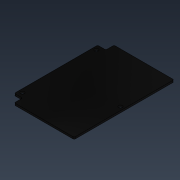
# Autodesk Inventor part: Base Station PCB
Saved by Autodesk Inventor 2022.1 (Build 261234020, 234B)
## iProperties
Created: 2017-10-12
Part Number: Base Station PCB
Material: Phenolharz
Document SubType Name: Modeling
Designer: ryll
Density: 1.38 g/cm^3
Appearance: Glänzend - Schwarz
Mass: 15.8976 g
Surface Area: 149.895 cm^2
Volume: 11.52 cm^3
Author: ryll
Autodesk Inventor part; units mm, degrees
ref_plane "YZ Plane" through (0, 0, 0) normal (1, 0, 0) x (0, 1, 0)
ref_plane "XZ Plane" through (0, 0, 0) normal (0, 1, 0) x (-1, 0, 0)
ref_plane "XY Plane" through (0, 0, 0) normal (0, 0, 1) x (1, 0, 0)
sketch "Skizze1" plane through (0, 0, 0) normal (0, 0, 1) x (1, 0, 0)
  line L0 (-22, -42.5) -> (29, -42.5)
  line L1 (29, -42.5) -> (29, 42.5)
  line L2 (29, 42.5) -> (-22, 42.5)
  line L3 (-29, 35.5) -> (-29, -35.5)
  line L4 (-22, -42.5) -> (-22, -35.5)
  line L5 (-22, -35.5) -> (-29, -35.5)
  line L6 (-22, 42.5) -> (-22, 35.5)
  line L7 (-22, 35.5) -> (-29, 35.5)
  line L8 (0, 59.5) -> (0, -59.5) projected
  line L9 (-40.6, 0) -> (40.6, 0) projected
  dimension "d22" = 58
  dimension "d23" = 85
  dimension "d24" = 7
  dimension "d25" = 7
  dimension "d26" = 7
  dimension "d27" = 7
  constraints: 16 end point, 3 horizontal, 2 parallel, 2 vertical, 1 perpendicular, 2 other
  measures "d22" distance between parallel lines of L1 L3
  measures "d23" distance of L0.end L1.end
  measures "d24" distance of L6.end L3.start
  measures "d25" distance of L2.end L6.end
  measures "d26" distance of L4.end L3.end
  measures "d27" distance of L0.start L4.end
extrude "Extrusion1" add sketch "Skizze1" along normal blind 1.6
sketch "Skizze2" plane through (0, 0, 1.6) normal (0, 0, 1) x (1, 0, 0)
  line L0 (-22, -42.5) -> (29, -42.5) projected
  line L1 (29, -42.5) -> (29, 42.5) projected
  line L2 (29, 42.5) -> (-22, 42.5) projected
  line L3 (-29, 35.5) -> (-29, -35.5) projected
  line L4 (-22, 42.5) -> (-22, 35.5) projected
  line L5 (-22, 35.5) -> (-29, 35.5) projected
  line L6 (-29, -35.5) -> (-22, -35.5) projected
  line L7 (-22, -35.5) -> (-22, -42.5) projected
  line L8 (-40.6, 0) -> (40.6, 0) projected
  point P0 (0, 0)
  point P1 (-26, 31.5)
  point P2 (-26, -31.5)
  point P3 (26, 0)
  dimension "d28" = 55
  dimension "d29" = 11
  dimension "d30" = 3
  dimension "d31" = 3
  dimension "d32" = 11
  constraints: 1 point on line
  measures "d28" distance from line of point (26, 0) L3
  measures "d29" distance from line of point (-26, -31.5) L0
  measures "d30" distance from line of L3 point (-26, -31.5)
  measures "d31" distance from line of L3 point (-26, 31.5)
  measures "d32" distance from line of L2 point (-26, 31.5)
hole "Bohrung1" at (-26, 31.5, 1.6) at (-26, -31.5, 1.6) at (26, 0, 1.6) direction (0, 0, -1) diameter 3.2 end through all
fillet "Rundung1" radius 1 8 edges at (29, -42.5, 0.8) (29, 42.5, 0.8) (-22, -35.5, 0.8) (-22, -42.5, 0.8) (-29, -35.5, 0.8) (-29, 35.5, 0.8) (-22, 35.5, 0.8) (-22, 42.5, 0.8)
equation "\"d26\" = d24"
equation "\"d27\" = d25"
